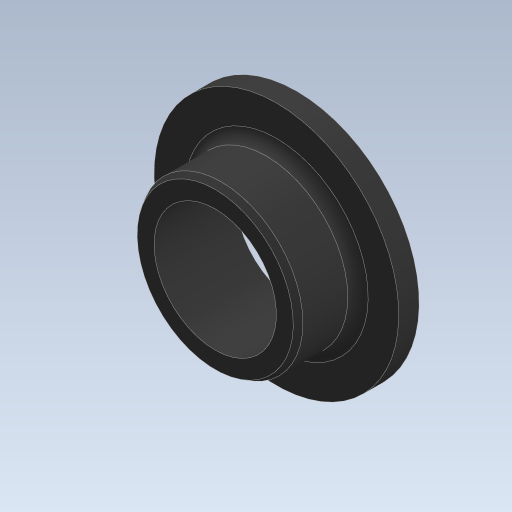
# Autodesk Inventor part: _GFM-0608-04
Saved by Autodesk Inventor 2024 (Build 280153000, 153)
## iProperties
Created: 2023-09-16
Part Number: _GFM-0608-04
Material: アセタール樹脂、黒
Document SubType Name: Modeling
Designer: michi
Density: 1.425 g/cm^3
Appearance: ゴム - 黒
Author: michi
Autodesk Inventor part; units mm, degrees
ref_plane "YZ Plane" through (0, 0, 0) normal (1, 0, 0) x (0, 1, 0)
ref_plane "XZ Plane" through (0, 0, 0) normal (0, 1, 0) x (-1, 0, 0)
ref_plane "XY Plane" through (0, 0, 0) normal (0, 0, 1) x (1, 0, 0)
sketch "スケッチ1" plane through (0, 0, 0) normal (1, 0, 0) x (0, 1, 0)
  line L0 (0, -0.8) -> (0, 4.8) construction
  line L1 (3, 4) -> (4, 4)
  line L2 (4, 4) -> (4, 1)
  line L3 (4, 1) -> (3, 1)
  line L4 (3, 1) -> (3, 4)
  line L5 (3, 1) -> (6, 1)
  line L6 (6, 1) -> (6, 0)
  line L7 (6, 0) -> (3, 0)
  line L8 (3, 0) -> (3, 1)
  point P0 (0, 0)
  point P1 (4, 1)
  dimension "d0" = 6
  dimension "d1" = 8
  dimension "d2" = 1
  dimension "d3" = 4
  dimension "d4" = 12
  constraints: 16 end point, 4 parallel, 2 horizontal, 2 perpendicular, 1 point on line
  measures "d0" diameter of L4 L0
  measures "d1" diameter of L2 L0
  measures "d2" distance of L5.end L6.end
  measures "d3" distance between parallel lines of L7 L1
  measures "d4" diameter of L6 L0
revolve "回転1" add sketch "スケッチ1" angle 360 about axis through (0, 0, -10) along (0, 0, 1)
fillet "フィレット1" radius 0.5 1 edges at (0, -4, 1)
chamfer "面取り1" distance 0.3 angle 30 1 edges at (0, -4, 4) measured on face at (0.3219, 3.987, 2.3333)
